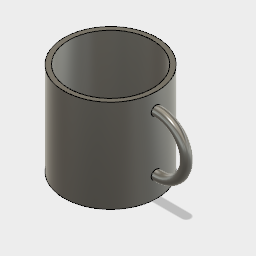
cup (Autodesk Fusion 360 design; units mm, degrees)
Autodesk Fusion 360 part; units mm, degrees
cylinder "圆柱体基本要素1" add diameter 20 height 20 placed x (1, 0, 0) y (0, 0, -1) z (0, 1, 0) at (0, 0, 0) makes body 1
torus "圆环体基本要素2" add centre line diameter 12 section diameter 2 placed x (1, 0, 0) y (0, 1, 0) z (0, 0, 1) at (26, 29, 0) separate body makes body 2
move_body "MoveFace2" bodies 2 to x (1, 0, 0) y (0, 1, 0) z (0, 0, 1) at (-15.5114, -18.4777, 0.1779) on bodies 2
combine "合并1" operation add target body 1 tool bodies 2
shell "抽壳1" thickness 1 removed faces 1 at (2.3712, 20, 3.5556) on bodies 1
cylinderprimitive "圆柱体基本要素2" [rolled back] height 20 diameter 18
torusprimitive "圆环体基本要素1" [rolled back] minor diameter 2 major diameter 12.166
moveface "MoveFace1" [rolled back]
